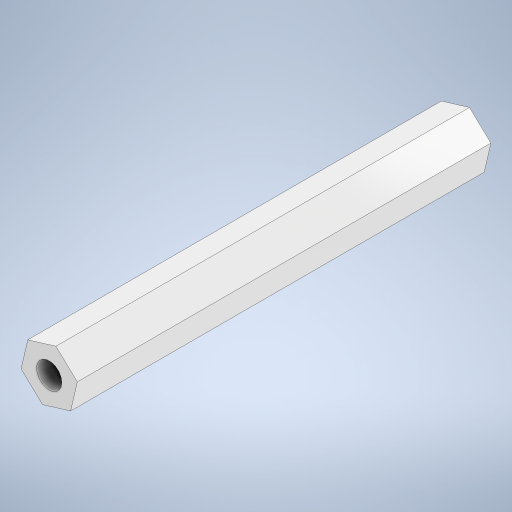
# Autodesk Inventor part: стойка
Saved by Autodesk Inventor 2023 (Build 270158000, 158)
## iProperties
Created: 2024-03-01
Part Number: стойка
Material: Типовые
Document SubType Name: Modeling
Designer: liza
Density: 1 g/cm^3
Appearance: По умолчанию
Author: liza
Autodesk Inventor part; units mm, degrees
ref_plane "YZ Plane" through (0, 0, 0) normal (1, 0, 0) x (0, 1, 0)
ref_plane "XZ Plane" through (0, 0, 0) normal (0, 1, 0) x (-1, 0, 0)
ref_plane "XY Plane" through (0, 0, 0) normal (0, 0, 1) x (1, 0, 0)
sketch "Эскиз1" plane through (0, 0, 0) normal (0, 0, 1) x (1, 0, 0)
  line L0 (4.4225, 1.3322) -> (3.365, -3.1639)
  line L1 (3.365, -3.1639) -> (-1.0575, -4.4961)
  line L2 (-1.0575, -4.4961) -> (-4.4225, -1.3322)
  line L3 (-4.4225, -1.3322) -> (-3.365, 3.1639)
  line L4 (-3.365, 3.1639) -> (1.0575, 4.4961)
  line L5 (1.0575, 4.4961) -> (4.4225, 1.3322)
  circle A0 centre (0, 0) radius 2
  point P0 (-1.1537, 3.83)
  dimension "d0" = 8
  dimension "d1" = 7.66
  dimension "d2" = 4
  constraints: 12 end point, 2 coincident, 1 centre point, 1 midpoint, 13 other
  measures "d0" distance from line of L1 point (-1.154, 3.83)
  measures "d1" vertical distance of L0.end L4.end
  measures "d2" diameter of A0
extrude "Выдавливание1" add sketch "Эскиз1" along normal blind 65
